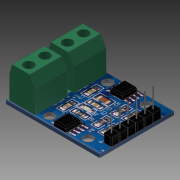
# Autodesk Inventor part: L9110S 모터 드라이버
Saved by Autodesk Inventor 2015 (Build 190159000, 159)
## iProperties
Created: 2018-01-06
Part Number: L9110S 모터 드라이버
Material: 일반
Document SubType Name: Modeling
Designer: choi jong in
Density: 1 g/cm^3
Appearance: 기본값
Author: choi jong in
Autodesk Inventor part; units mm, degrees
ref_plane "YZ Plane" through (0, 0, 0) normal (1, 0, 0) x (0, 1, 0)
ref_plane "XZ Plane" through (0, 0, 0) normal (0, 1, 0) x (-1, 0, 0)
ref_plane "XY Plane" through (0, 0, 0) normal (0, 0, 1) x (1, 0, 0)
sketch "스케치1" plane through (0, 0, 0) normal (0, 1, 0) x (-1, 0, 0)
  line L0 (-14.5, 11.5) -> (14.5, 11.5)
  line L1 (14.5, 11.5) -> (14.5, -11.5)
  line L2 (14.5, -11.5) -> (-14.5, -11.5)
  line L3 (-14.5, -11.5) -> (-14.5, 11.5)
  line L4 (-14.5, 11.5) -> (14.5, -11.5) construction
  line L5 (14.5, 11.5) -> (-14.5, -11.5) construction
  point P0 (0, 0)
  dimension "d0" = 29
  dimension "d1" = 23
  constraints: 12 end point, 2 midpoint, 2 parallel, 1 horizontal, 1 perpendicular
  measures "d0" distance of L1.end L2.end
  measures "d1" distance of L0.end L1.end
extrude "돌출1" add sketch "스케치1" along normal blind 1
sketch "스케치2" plane through (0, 1, 0) normal (0, 1, 0) x (1, 0, 0)
  line L0 (14.5, -11.5) -> (14.5, 11.5) projected
  point P0 (0, 0)
  point P1 (8.5, 9)
  dimension "d4" = 6
  dimension "d5" = 9
  measures "d4" distance from line of L0 point (8.5, 9)
  measures "d5" vertical distance of point (8.5, 9) point (0, 0)
hole "구멍1" at (8.5, 1, -9) direction (0, -1, 0) diameter 3 end through all
pattern_linear "직사각형 패턴1" count 2 spacing 18 along (0, 0, 1) count 2 spacing 12 along (-1, 0, 0) of "구멍1"
sketch "스케치3" plane through (0, 1, 0) normal (0, 1, 0) x (1, 0, 0)
  line L0 (11.9, -7.75) -> (14.4, -7.75) construction
  line L1 (14.4, -7.75) -> (14.4, 7.75) construction
  line L2 (14.4, 7.75) -> (11.9, 7.75) construction
  line L3 (11.9, 7.75) -> (11.9, -7.75) construction
  line L4 (11.9, -7.75) -> (14.4, 7.75) construction
  line L5 (14.4, -7.75) -> (11.9, 7.75) construction
  line L6 (14.4, -7.75) -> (11.9, -7.75)
  line L7 (11.9, -7.75) -> (11.9, -5.25)
  line L8 (11.9, -5.25) -> (14.4, -5.25)
  line L9 (14.4, -5.25) -> (14.4, -7.75)
  line L10 (14.5, -11.5) -> (14.5, 11.5) projected
  line L11 (0, 0) -> (13.15, 0) construction
  dimension "d19" = 2.5
  dimension "d20" = 15.5
  dimension "d21" = 2.5
  dimension "d22" = 2.6
  constraints: 22 end point, 4 parallel, 3 horizontal, 2 midpoint, 2 perpendicular, 1 point on line
  measures "d19" distance of L2.end L1.end
  measures "d20" distance of L1.end L0.end
  measures "d21" distance of L6.end L7.end
  measures "d22" distance between parallel lines of L10 L3
extrude "돌출2" add sketch "스케치3" along normal blind 2.5
chamfer "모따기1" distance 0.2 angle 45 4 edges at (14.4, 2.25, 7.75) (14.4, 2.25, 5.25) (11.9, 2.25, 7.75) (11.9, 2.25, 5.25)
sketch "스케치4" plane through (0, 3.5, 0) normal (0, 1, 0) x (1, 0, 0)
  line L0 (11.9, -5.45) -> (12.1, -5.25) construction
  line L1 (11.9, -5.45) -> (11.9, -7.55) construction
  line L2 (12.1, -7.75) -> (11.9, -7.55) construction
  line L3 (12.1, -7.75) -> (14.2, -7.75) construction
  line L4 (14.4, -7.55) -> (14.2, -7.75) construction
  line L5 (14.4, -7.55) -> (14.4, -5.45) construction
  line L6 (14.2, -5.25) -> (14.4, -5.45) construction
  line L7 (14.2, -5.25) -> (12.1, -5.25) construction
  line L8 (11.9, -6.5) -> (14.4, -6.5) construction
  line L9 (13.15, -7.75) -> (13.15, -5.25) construction
  line L10 (13.25, -6.6) -> (13.05, -6.6)
  line L11 (13.05, -6.6) -> (13.05, -6.4)
  line L12 (13.05, -6.4) -> (13.25, -6.4)
  line L13 (13.25, -6.4) -> (13.25, -6.6)
  line L14 (13.25, -6.6) -> (13.05, -6.4) construction
  line L15 (13.05, -6.6) -> (13.25, -6.4) construction
  point P0 (0, 0)
  point P1 (13.15, -6.5)
  dimension "d28" = 0.2
  dimension "d29" = 0.2
  constraints: 16 end point, 7 midpoint, 2 parallel, 1 horizontal, 1 perpendicular
  measures "d28" distance of L11.end L12.end
  measures "d29" distance of L10.end L11.end
extrude "돌출3" add sketch "스케치4" along normal blind 6 and the other way blind 4
chamfer "모따기2" distance 0.05 angle 45 8 edges at (13.25, 9.5, 6.5) (13.15, 9.5, 6.4) (13.05, 9.5, 6.5) (13.15, 9.5, 6.6) (13.25, -0.5, 6.5) (13.15, -0.5, 6.6) (13.05, -0.5, 6.5) (13.15, -0.5, 6.4)
pattern_linear "직사각형 패턴2" count 6 spacing 2.6 along (0, 0, -1) of "돌출2", "모따기1", "돌출3", "모따기2"
sketch "스케치5" plane through (0, 1, 0) normal (0, 1, 0) x (1, 0, 0)
  line L0 (11.9, 7.55) -> (12.1, 7.75) projected
  line L1 (14.2, 7.75) -> (12.1, 7.75) projected
  line L2 (12.1, -7.75) -> (14.2, -7.75) projected
  line L3 (12.1, 7.75) -> (14.2, 7.75)
  line L4 (14.2, 7.75) -> (14.2, -7.75)
  line L5 (14.2, -7.75) -> (12.1, -7.75)
  line L6 (12.1, -7.75) -> (12.1, 7.75)
  point P0 (0, 0)
  dimension "d40" = 15.5
  constraints: 8 end point, 2 parallel, 1 horizontal, 1 perpendicular
  measures "d40" distance of L3.end L2.end
extrude "돌출4" add sketch "스케치5" along normal blind 2.4
sketch "스케치6" plane through (0, 1, 0) normal (0, 1, 0) x (1, 0, 0)
  line L0 (-0.2, -11) -> (3.5, -11)
  line L1 (3.5, -11) -> (3.5, -6.5)
  line L2 (3.5, -6.5) -> (-0.2, -6.5)
  line L3 (-0.2, -6.5) -> (-0.2, -11)
  line L4 (14.5, -11.5) -> (14.5, 11.5) projected
  line L5 (-14.5, -11.5) -> (14.5, -11.5) projected
  line L6 (0, 0) -> (-15.3951, 0) construction
  line L7 (-0.2, 11) -> (3.5, 11)
  line L8 (3.5, 11) -> (3.5, 6.5)
  line L9 (3.5, 6.5) -> (-0.2, 6.5)
  line L10 (-0.2, 6.5) -> (-0.2, 11)
  dimension "d43" = 4.5
  dimension "d44" = 3.7
  dimension "d45" = 11
  dimension "d46" = 0.5
  constraints: 18 end point, 4 symmetric about line, 2 horizontal, 2 parallel, 1 perpendicular
  measures "d43" distance of L0.end L1.end
  measures "d44" distance of L1.end L2.end
  measures "d45" distance between parallel lines of L4 L1
  measures "d46" distance between parallel lines of L5 L0
extrude "돌출5" add sketch "스케치6" along normal blind 1.5
chamfer "모따기3" distance 0.5 angle 30 1 edges at (3.5, 2.5, 8.75) measured on face at (3.5, 1.5, 9.5)
chamfer "모따기4" distance 0.5 angle 30 1 edges at (1.5057, 2.5, 11) measured on face at (2.1704, 1.5, 11)
chamfer "모따기5" distance 0.5 angle 30 1 edges at (-0.2, 2.5, 8.6057) measured on face at (-0.2, 1.5, 9.4038)
chamfer "모따기6" distance 0.5 angle 30 1 edges at (1.65, 2.5, 6.5) measured on face at (2.1704, 1.5, 6.5)
chamfer "모따기7" distance 0.5 angle 30 1 edges at (1.65, 2.5, -6.5) measured on face at (2.2667, 1.5, -6.5)
chamfer "모따기8" distance 0.5 angle 30 1 edges at (-0.2, 2.5, -8.8943) measured on face at (-0.2, 1.5, -8.0962)
chamfer "모따기9" distance 0.5 angle 30 1 edges at (3.5, 2.5, -8.8943) measured on face at (3.5, 1.5, -8.0962)
chamfer "모따기10" distance 0.5 angle 30 1 edges at (1.65, 2.5, -11) measured on face at (2.1704, 1.5, -11)
sketch "스케치7" plane through (0, 1, 0) normal (0, 1, 0) x (1, 0, 0)
  line L0 (-14, -11) -> (-6, -11)
  line L1 (-6, -11) -> (-6, -1)
  line L2 (-6, -1) -> (-14, -1)
  line L3 (-14, -1) -> (-14, -11)
  line L4 (14.5, -11.5) -> (-14.5, -11.5) projected
  line L5 (-14.5, 11.5) -> (-14.5, -11.5) projected
  point P0 (0, 0)
  dimension "d73" = 8
  dimension "d74" = 10
  dimension "d75" = 0.5
  dimension "d76" = 0.5
  constraints: 8 end point, 2 parallel, 1 horizontal, 1 perpendicular
  measures "d73" distance of L2.end L1.end
  measures "d74" distance of L1.end L0.end
  measures "d75" distance between parallel lines of L4 L0
  measures "d76" distance between parallel lines of L5 L3
extrude "돌출6" add sketch "스케치7" along normal blind 10
chamfer "모따기11" distance 3 angle 15 1 edges at (-14, 11, 6) measured on face at (-14, 4.3333, 4.3333)
chamfer "모따기12" distance 3 angle 30 1 edges at (-6, 11, 6) measured on face at (-6, 4.3333, 7.6667)
mirror "대칭1" about plane through (0, 0, 0) normal (0, 0, 1) of "돌출6", "모따기11", "모따기12"
sketch "스케치8" plane through (0, 1, 0) normal (0, 1, 0) x (1, 0, 0)
  line L0 (-14, 11) -> (-6, 11) projected
  line L1 (-6, 11) -> (-6, 1) projected
  line L2 (-6, 1) -> (-14, 1) projected
  line L3 (-14, 1) -> (-14, 11) projected
  line L4 (-14, -11) -> (-14, -1) projected
  line L5 (-14, -1) -> (-6, -1) projected
  line L6 (-6, -1) -> (-6, -11) projected
  line L7 (-6, -11) -> (-14, -11) projected
  line L8 (-0.2, -11) -> (-0.2, -6.5) projected
  line L9 (-0.2, -6.5) -> (3.5, -6.5) projected
  line L10 (3.5, -6.5) -> (3.5, -11) projected
  line L11 (3.5, -11) -> (-0.2, -11) projected
  line L12 (3.5, 11) -> (3.5, 6.5) projected
  line L13 (3.5, 6.5) -> (-0.2, 6.5) projected
  line L14 (-0.2, 6.5) -> (-0.2, 11) projected
  line L15 (-0.2, 11) -> (3.5, 11) projected
  line L16 (-14.5, -11.5) -> (14.5, -11.5) projected
  line L17 (14.5, -11.5) -> (14.5, 11.5) projected
  line L18 (14.5, 11.5) -> (-14.5, 11.5) projected
  line L19 (-14.5, 11.5) -> (-14.5, -11.5) projected
  circle A0 centre (8.5, 9) radius 1.5 projected
  circle A1 centre (8.5, -9) radius 1.5 projected
  circle A2 centre (-3.5, 9) radius 1.5 projected
  circle A3 centre (-3.5, -9) radius 1.5 projected
  line L20 (14.2, 5.25) -> (14.2, 5.15) projected
  line L21 (14.4, 4.95) -> (14.2, 5.15) projected
  line L22 (14.4, 4.95) -> (14.4, 2.85) projected
  line L23 (14.2, 2.65) -> (14.4, 2.85) projected
  line L24 (14.2, 2.65) -> (14.2, 2.55) projected
  line L25 (14.4, 2.35) -> (14.2, 2.55) projected
  line L26 (14.4, 2.35) -> (14.4, 0.25) projected
  line L27 (14.2, 0.05) -> (14.4, 0.25) projected
  line L28 (14.2, 0.05) -> (14.2, -0.05) projected
  line L29 (14.4, -0.25) -> (14.2, -0.05) projected
  line L30 (14.4, -0.25) -> (14.4, -2.35) projected
  line L31 (14.2, -2.55) -> (14.4, -2.35) projected
  line L32 (14.2, -2.55) -> (14.2, -2.65) projected
  line L33 (14.4, -2.85) -> (14.2, -2.65) projected
  line L34 (14.4, -2.85) -> (14.4, -4.95) projected
  line L35 (14.2, -5.15) -> (14.4, -4.95) projected
  line L36 (14.2, -5.15) -> (14.2, -5.25) projected
  line L37 (14.4, -5.45) -> (14.2, -5.25) projected
  line L38 (14.4, -5.45) -> (14.4, -7.55) projected
  line L39 (14.2, -7.75) -> (14.4, -7.55) projected
  line L40 (14.2, -7.75) -> (12.1, -7.75) projected
  line L41 (11.9, -7.55) -> (12.1, -7.75) projected
  line L42 (11.9, -7.55) -> (11.9, -5.45) projected
  line L43 (12.1, -5.25) -> (11.9, -5.45) projected
  line L44 (12.1, -5.25) -> (12.1, -5.15) projected
  line L45 (11.9, -4.95) -> (12.1, -5.15) projected
  line L46 (11.9, -4.95) -> (11.9, -2.85) projected
  line L47 (12.1, -2.65) -> (11.9, -2.85) projected
  line L48 (12.1, -2.65) -> (12.1, -2.55) projected
  line L49 (11.9, -2.35) -> (12.1, -2.55) projected
  line L50 (11.9, -2.35) -> (11.9, -0.25) projected
  line L51 (12.1, -0.05) -> (11.9, -0.25) projected
  line L52 (12.1, -0.05) -> (12.1, 0.05) projected
  line L53 (11.9, 0.25) -> (12.1, 0.05) projected
  line L54 (11.9, 0.25) -> (11.9, 2.35) projected
  line L55 (12.1, 2.55) -> (11.9, 2.35) projected
  line L56 (12.1, 2.55) -> (12.1, 2.65) projected
  line L57 (11.9, 2.85) -> (12.1, 2.65) projected
  line L58 (11.9, 2.85) -> (11.9, 4.95) projected
  line L59 (12.1, 5.15) -> (11.9, 4.95) projected
  line L60 (12.1, 5.15) -> (12.1, 5.25) projected
  line L61 (11.9, 5.45) -> (12.1, 5.25) projected
  line L62 (11.9, 5.45) -> (11.9, 7.55) projected
  line L63 (12.1, 7.75) -> (11.9, 7.55) projected
  line L64 (12.1, 7.75) -> (14.2, 7.75) projected
  line L65 (14.4, 7.55) -> (14.2, 7.75) projected
  line L66 (14.4, 7.55) -> (14.4, 5.45) projected
  line L67 (14.2, 5.25) -> (14.4, 5.45) projected
  line L68 (14.5347, -11) -> (-14.5, -11) construction
  line L69 (-14.5, -11) -> (-14.5, 11.9646) construction
  line L70 (-14.5, 11.9646) -> (14.5347, 11.9646) construction
  line L71 (14.5347, 11.9646) -> (14.5347, -11) construction
  point P0 (0, 0)
  constraints: 2 point on line, 1 horizontal, 2 other
decal "전사1"
sketch "스케치10" plane through (-14, 1, -11) normal (-1, 0, 0) x (0, 0, 1)
  line L0 (0.5, 6.5) -> (4.5, 6.5)
  line L1 (4.5, 6.5) -> (4.5, 0.5)
  line L2 (4.5, 0.5) -> (0.5, 0.5)
  line L3 (0.5, 0.5) -> (0.5, 6.5)
  line L4 (5.5, 6.5) -> (9.5, 6.5)
  line L5 (9.5, 6.5) -> (9.5, 0.5)
  line L6 (9.5, 0.5) -> (5.5, 0.5)
  line L7 (5.5, 0.5) -> (5.5, 6.5)
  line L8 (12.5, 6.5) -> (16.5, 6.5)
  line L9 (16.5, 6.5) -> (16.5, 0.5)
  line L10 (16.5, 0.5) -> (12.5, 0.5)
  line L11 (12.5, 0.5) -> (12.5, 6.5)
  line L12 (17.5, 6.5) -> (21.5, 6.5)
  line L13 (21.5, 6.5) -> (21.5, 0.5)
  line L14 (21.5, 0.5) -> (17.5, 0.5)
  line L15 (17.5, 0.5) -> (17.5, 6.5)
  line L16 (0, 0) -> (0, 7) projected
  line L17 (10, 7) -> (0, 7) projected
  line L18 (10, 0) -> (0, 0) projected
  line L19 (10, 0) -> (10, 7) projected
  line L20 (12, 0) -> (12, 7) projected
  line L21 (22, 0) -> (22, 7) projected
  point P0 (11, -1)
  dimension "d136" = 0.5
  dimension "d137" = 0.5
  dimension "d138" = 0.5
  dimension "d139" = 0.5
  dimension "d140" = 4
  dimension "d141" = 4
  dimension "d142" = 4
  dimension "d143" = 4
  dimension "d144" = 0.5
  dimension "d145" = 0.5
  constraints: 32 end point, 8 parallel, 6 point on line, 4 horizontal, 4 perpendicular
  measures "d136" distance between parallel lines of L16 L3
  measures "d137" distance between parallel lines of L0 L17
  measures "d138" distance between parallel lines of L18 L2
  measures "d139" distance between parallel lines of L19 L5
  measures "d140" distance of L1.end L2.end
  measures "d141" distance of L5.end L6.end
  measures "d142" distance of L9.end L10.end
  measures "d143" distance of L13.end L14.end
  measures "d144" distance between parallel lines of L20 L11
  measures "d145" distance between parallel lines of L21 L13
extrude "돌출8" cut sketch "스케치10" against normal blind 7 contours L0 L1 L2 L3 | L4 L5 L6 L7 | L8 L9 L10 L11 | L12 L13 L14 L15
sketch "스케치9" plane through (0, 11, 0) normal (0, 1, 0) x (1, 0, 0)
  circle A0 centre (-10.4641, -8.5) radius 1.5
  circle A1 centre (-10.4641, -3.5) radius 1.5
  circle A2 centre (-10.4641, 3.5) radius 1.5
  circle A3 centre (-10.4641, 8.5) radius 1.5
  line L0 (-13.1962, -11) -> (-7.7321, -11) construction
  line L1 (-10.4641, -11) -> (-10.4641, 11.3401) construction
  line L2 (-7.7321, -1) -> (-13.1962, -1) projected
  line L3 (-7.7321, 1) -> (-13.1962, 1) projected
  line L4 (-13.1962, 11) -> (-7.7321, 11) projected
  point P0 (0, 0)
  dimension "d129" = 3
  dimension "d130" = 2.5
  dimension "d131" = 2.5
  dimension "d132" = 2.5
  dimension "d133" = 2.5
  constraints: 4 centre point, 4 point on line, 3 equal radius, 2 end point, 1 midpoint, 1 vertical
  measures "d129" diameter of A0
  measures "d130" distance from line of L0 A0.centre
  measures "d131" distance from line of L2 A1.centre
  measures "d132" distance from line of A2.centre L3
  measures "d133" distance from line of A3.centre L4
sketch "스케치11" plane through (-7, 1, 0) normal (-1, 0, 0) x (0, 1, 0)
  line L0 (6, 10) -> (1, 10)
  line L1 (1, 10) -> (1, 7)
  line L2 (1, 7) -> (6, 7)
  line L3 (6, 7) -> (6, 10)
  line L4 (6, 5) -> (1, 5)
  line L5 (1, 5) -> (1, 2)
  line L6 (1, 2) -> (6, 2)
  line L7 (6, 2) -> (6, 5)
  line L8 (6, -2) -> (1, -2)
  line L9 (1, -2) -> (1, -5)
  line L10 (1, -5) -> (6, -5)
  line L11 (6, -5) -> (6, -2)
  line L12 (6, -7) -> (1, -7)
  line L13 (1, -7) -> (1, -10)
  line L14 (1, -10) -> (6, -10)
  line L15 (6, -10) -> (6, -7)
  line L16 (0.5, 10.5) -> (6.5, 10.5) projected
  line L17 (6.5, 6.5) -> (0.5, 6.5) projected
  line L18 (0.5, 6.5) -> (0.5, 10.5) projected
  line L19 (0.5, 5.5) -> (6.5, 5.5) projected
  line L20 (6.5, 1.5) -> (0.5, 1.5) projected
  line L21 (0.5, -1.5) -> (6.5, -1.5) projected
  line L22 (6.5, -5.5) -> (0.5, -5.5) projected
  line L23 (0.5, -6.5) -> (6.5, -6.5) projected
  line L24 (6.5, -10.5) -> (0.5, -10.5) projected
  line L25 (6.5, 10.5) -> (6.5, 6.5) projected
  line L26 (0.5, 10.5) -> (6.5, 10.5) projected
  line L27 (0.5, 6.5) -> (0.5, 10.5) projected
  line L28 (6.5, 6.5) -> (0.5, 6.5) projected
  line L29 (6.5, 5.5) -> (6.5, 1.5) projected
  line L30 (0.5, 5.5) -> (6.5, 5.5) projected
  line L31 (0.5, 1.5) -> (0.5, 5.5) projected
  line L32 (6.5, 1.5) -> (0.5, 1.5) projected
  line L33 (6.5, -1.5) -> (6.5, -5.5) projected
  line L34 (0.5, -1.5) -> (6.5, -1.5) projected
  line L35 (0.5, -5.5) -> (0.5, -1.5) projected
  line L36 (6.5, -5.5) -> (0.5, -5.5) projected
  line L37 (6.5, -6.5) -> (6.5, -10.5) projected
  line L38 (0.5, -6.5) -> (6.5, -6.5) projected
  line L39 (0.5, -10.5) -> (0.5, -6.5) projected
  line L40 (6.5, -10.5) -> (0.5, -10.5) projected
  point P0 (-1, 0)
  dimension "d149" = 0.5
  dimension "d150" = 0.5
  dimension "d151" = 0.5
  dimension "d152" = 0.5
  dimension "d153" = 0.5
  dimension "d154" = 0.5
  dimension "d155" = 0.5
  dimension "d156" = 0.5
  dimension "d157" = 0.5
  dimension "d160" = 0.5
  constraints: 32 end point, 8 parallel, 6 point on line, 4 horizontal, 4 perpendicular
  measures "d149" distance between parallel lines of L16 L0
  measures "d150" distance between parallel lines of L17 L2
  measures "d151" distance between parallel lines of L18 L1
  measures "d152" distance between parallel lines of L19 L4
  measures "d153" distance between parallel lines of L20 L6
  measures "d154" distance between parallel lines of L21 L8
  measures "d155" distance between parallel lines of L22 L10
  measures "d156" distance between parallel lines of L23 L12
  measures "d157" distance between parallel lines of L24 L14
  measures "d160" distance between parallel lines of L25 L3
extrude "돌출9" add sketch "스케치11" along normal blind 6
extrude "돌출10" cut sketch "스케치9" against normal up to surface (9 mm away)
sketch "스케치12" plane through (-13, 7, -10) normal (0, -1, 0) x (1, 0, 0)
  line L0 (0, 0) -> (0.2, 0)
  line L1 (0.2, 0) -> (0.2, 3)
  line L2 (0.2, 3) -> (0, 3)
  line L3 (0, 3) -> (0, 0)
  line L4 (0, 5) -> (0.2, 5)
  line L5 (0.2, 5) -> (0.2, 8)
  line L6 (0.2, 8) -> (0, 8)
  line L7 (0, 8) -> (0, 5)
  line L8 (0, 12) -> (0.2, 12)
  line L9 (0.2, 12) -> (0.2, 15)
  line L10 (0.2, 15) -> (0, 15)
  line L11 (0, 15) -> (0, 12)
  line L12 (0, 17) -> (0.2, 17)
  line L13 (0.2, 17) -> (0.2, 20)
  line L14 (0.2, 20) -> (0, 20)
  line L15 (0, 20) -> (0, 17)
  line L16 (0, -0.5) -> (0, 3.5) projected
  line L17 (-1, -0.5) -> (0, -0.5) projected
  line L18 (-1, 3.5) -> (0, 3.5) projected
  line L19 (-1, 4.5) -> (0, 4.5) projected
  line L20 (-1, 8.5) -> (0, 8.5) projected
  line L21 (-1, 11.5) -> (0, 11.5) projected
  line L22 (-1, 15.5) -> (0, 15.5) projected
  line L23 (-1, 16.5) -> (0, 16.5) projected
  line L24 (-1, 20.5) -> (0, 20.5) projected
  line L25 (2.5359, 0) -> (0, 0) projected
  line L26 (2.5359, 3) -> (0, 3) projected
  line L27 (2.5359, 5) -> (0, 5) projected
  line L28 (2.5359, 8) -> (0, 8) projected
  line L29 (2.5359, 12) -> (0, 12) projected
  line L30 (2.5359, 15) -> (0, 15) projected
  line L31 (2.5359, 17) -> (0, 17) projected
  line L32 (2.5359, 20) -> (0, 20) projected
  point P0 (13, 10)
  dimension "d163" = 0.2
  constraints: 32 end point, 9 collinear, 8 parallel, 6 point on line, 4 horizontal, 4 perpendicular
  measures "d163" distance between parallel lines of L1 L3
sketch "스케치13" plane through (-7, 2, -10) normal (0, 0, 1) x (1, 0, 0)
  line L0 (-6, -0.5) -> (-6, 5.5) construction
  line L1 (-7, -0.5) -> (-6, -0.5) construction
  line L2 (-6, 5.5) -> (-6.2737, 3.9478)
  line L3 (-5.2233, 1.8243) -> (-0.7321, -0.5)
  line L4 (-7, 5.5) -> (-6, 5.5) projected
  arc A0 (-6.2737, 3.9478) -> (-5.2233, 1.8243) centre (-4.3041, 3.6005) ccw
  line L5 (-0.7321, -0.5) -> (-0.7321, 9) construction
  point P0 (7, -2)
  point P1 (-6.529, 2.5)
  dimension "d167" = 10
  dimension "d169" = 3
  dimension "d170" = 2
  constraints: 6 end point, 3 point on line, 2 point on circle, 2 tangent, 1 centre point, 1 vertical
  measures "d167" angle of L0 L2
  measures "d169" distance from line of L4 point (-6.529, 2.5)
  measures "d170" radius of A0
sweep "스윕1" add profiles "스케치12" path "스케치13" path curves L2 A0 L3
